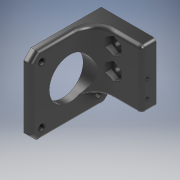
# Autodesk Inventor part: Y-Axis_Motor_Mount_LM3042
Saved by Autodesk Inventor 2020.3 (Build 243373000, 373)
## iProperties
Created: 2020-05-31
Part Number: Y-Axis_Motor_Mount_LM3042
Material: ABS Plastic
Document SubType Name: Modeling
Designer: rah75
Density: 1.06 g/cm^3
Appearance: Satin - Black
Author: rah75
Autodesk Inventor part; units mm, degrees
ref_plane "YZ Plane" through (0, 0, 0) normal (1, 0, 0) x (0, 1, 0)
ref_plane "XZ Plane" through (0, 0, 0) normal (0, 1, 0) x (-1, 0, 0)
ref_plane "XY Plane" through (0, 0, 0) normal (0, 0, 1) x (1, 0, 0)
sketch "Sketch1" plane through (0, 0, 0) normal (0, 0, 1) x (1, 0, 0)
  line L0 (-15, -21.15) -> (15, -21.15)
  line L1 (15, -21.15) -> (15, 21.15)
  line L2 (15, 21.15) -> (-15, 21.15)
  line L3 (-15, 21.15) -> (-15, -21.15)
  line L4 (-15, -21.15) -> (15, 21.15) construction
  line L5 (15, -21.15) -> (-15, 21.15) construction
  point P0 (0, 0)
  dimension "d0" = 30
  dimension "d1" = 42.3
  constraints: 12 end point, 2 midpoint, 2 parallel, 1 horizontal, 1 perpendicular
  measures "d0" distance of L2.end L1.end
  measures "d1" distance of L1.end L0.end
extrude "Extrusion1" add sketch "Sketch1" along normal blind 42.3
sketch "Sketch2" plane through (-15, 21.15, 0) normal (0, 1, 0) x (1, 0, 0)
  line L0 (30, 0) -> (0, 0) projected
  line L1 (0, 0) -> (0, -42.3) projected
  line L2 (30, -42.3) -> (0, -42.3) projected
  line L3 (30, 0) -> (30, -42.3) projected
  line L4 (4, -8) -> (30, -8)
  line L5 (30, -8) -> (30, -42.3)
  line L6 (30, -42.3) -> (4, -42.3)
  line L7 (4, -42.3) -> (4, -8)
  line L8 (4, -8) -> (30, -42.3) construction
  line L9 (30, -8) -> (4, -42.3) construction
  line L10 (30, 0) -> (30, -42.3) projected
  line L11 (30, -42.3) -> (0, -42.3) projected
  point P0 (15, 0)
  point P1 (17, -25.15)
  point P2 (4, -42.3)
  dimension "d4" = 8
  dimension "d5" = 4
  constraints: 12 end point, 2 collinear, 2 midpoint, 2 parallel, 1 horizontal, 1 perpendicular
  measures "d4" distance between parallel lines of L4 L0
  measures "d5" distance between parallel lines of L1 L7
extrude "Extrusion2" cut sketch "Sketch2" against normal through all contours L3 L2 L7 L4
sketch "Sketch3" plane through (-15, -21.15, 0) normal (-1, 0, 0) x (0, 0, 1)
  circle A0 centre (21.15, 21.15) radius 11.25
  line L0 (0, 42.3) -> (0, 0) projected
  line L1 (0, 42.3) -> (42.3, 42.3) projected
  point P0 (0, 21.15)
  point P1 (0, 21.15)
  point P2 (21.15, 42.3)
  dimension "d8" = 22.5
  constraints: 2 midpoint, 1 centre point, 1 horizontal alignment, 1 vertical alignment
  measures "d8" diameter of A0
extrude "Extrusion3" cut sketch "Sketch3" against normal blind 10
sketch "Sketch4" plane through (-11, 21.15, 42.3) normal (1, 0, 0) x (0, 0, -1)
  line L0 (5.65, -36.65) -> (36.65, -36.65) construction
  line L1 (36.65, -36.65) -> (36.65, -5.65) construction
  line L2 (36.65, -5.65) -> (5.65, -5.65) construction
  line L3 (5.65, -5.65) -> (5.65, -36.65) construction
  circle A0 centre (21.15, -21.15) radius 11.25 construction
  line L4 (5.65, -36.65) -> (36.65, -5.65) construction
  line L5 (36.65, -36.65) -> (5.65, -5.65) construction
  point P0 (42.3, -21.15)
  dimension "d11" = 31
  dimension "d12" = 31
  constraints: 12 end point, 4 coincident, 2 midpoint, 2 parallel, 1 horizontal, 1 perpendicular
  measures "d11" distance of L2.end L1.end
  measures "d12" distance of L1.end L0.end
hole "Hole1" at (-11, 15.5, 36.65) at (-11, -15.5, 36.65) at (-11, -15.5, 5.65) direction (-1, 0, 0) diameter 3.4 end through all start extended yes clearance for "Socket Head Cap Screw" size "M3" standard "Ansi Metric M Profile"
sketch "Sketch5" plane through (-11, 21.15, 8) normal (0, 0, 1) x (1, 0, 0)
  line L0 (0, 0) -> (0, -42.3) projected
  line L1 (26, -42.3) -> (0, -42.3) projected
  line L2 (26, 0) -> (26, -42.3) projected
  line L3 (0, -32.3) -> (26, -32.3)
  line L4 (26, -32.3) -> (26, -42.3)
  line L5 (26, -42.3) -> (0, -42.3)
  line L6 (0, -42.3) -> (0, -32.3)
  line L7 (0, -32.3) -> (26, -42.3) construction
  line L8 (26, -32.3) -> (0, -42.3) construction
  line L9 (0, 0) -> (26, 0) projected
  point P0 (11, -21.15)
  point P1 (13, -37.3)
  point P2 (0, -32.3)
  dimension "d21" = 10
  constraints: 12 end point, 2 midpoint, 2 parallel, 1 horizontal, 1 perpendicular
  measures "d21" distance between parallel lines of L3 L1
extrude "Extrusion4" cut sketch "Sketch5" against normal blind 10 contours L3 L2 L1 L0
fillet "Fillet2" radius 10 1 edges at (-11, 5, 8)
chamfer "Chamfer1" distance 4 angle 45 3 edges at (-13, 21.15, 42.3) (-13, -21.15, 42.3) (-13, -21.15, 0)
sketch "Sketch6" plane through (15, -11.15, 8) normal (0, 0, 1) x (1, 0, 0)
  line L0 (4.601, 32.6196) -> (1.0678, 32.6196)
  line L1 (1.0678, 32.6196) -> (1.0678, 6.6196)
  line L2 (1.0678, 6.6196) -> (4.601, 6.6196)
  line L3 (4.601, 6.6196) -> (4.601, 32.6196)
  line L4 (-16, 32.3) -> (0, 32.3) projected
  line L5 (-26, -6) -> (-26, 28.3) projected
  line L6 (-26, -10) -> (-26, -6) projected
  line L7 (0, 32.3) -> (0, 0) projected
  line L8 (-11.125, 22.9184) -> (-15.25, 20.5369)
  line L9 (-15.25, 20.5369) -> (-19.375, 22.9184)
  line L10 (-19.375, 22.9184) -> (-19.375, 27.6816)
  line L11 (-19.375, 27.6816) -> (-15.25, 30.0631)
  line L12 (-15.25, 30.0631) -> (-11.125, 27.6816)
  line L13 (-11.125, 27.6816) -> (-11.125, 22.9184)
  line L14 (-11.125, 10.9184) -> (-15.25, 8.5369)
  line L15 (-15.25, 8.5369) -> (-19.375, 10.9184)
  line L16 (-19.375, 10.9184) -> (-19.375, 15.6816)
  line L17 (-19.375, 15.6816) -> (-15.25, 18.0631)
  line L18 (-15.25, 18.0631) -> (-11.125, 15.6816)
  line L19 (-11.125, 15.6816) -> (-11.125, 10.9184)
  line L20 (-30, 28.3) -> (-30, -6) projected
  point P0 (-15, 11.15)
  point P1 (-15.25, 25.3)
  point P2 (-15.25, 13.3)
  point P3 (-15.25, 25.3)
  point P4 (-15.25, 13.3)
  dimension "d29" = 26
  dimension "d30" = 7
  dimension "d31" = 19
  dimension "d33" = 8.25
  dimension "d45" = 14.75
  constraints: 32 end point, 2 coincident, 2 parallel, 1 collinear, 1 horizontal, 1 perpendicular, 1 point on line, 1 vertical, 1 vertical alignment, 26 other
  measures "d29" distance of L1.end L0.end
  measures "d30" distance from line of L4 point (-15.25, 25.3)
  measures "d31" distance from line of L4 point (-15.25, 13.3)
  measures "d33" distance between parallel lines of L16 L19
  measures "d45" distance from line of L20 point (-15.25, 25.3)
extrude "Extrusion5" cut sketch "Sketch6" along normal blind 10 and the other way blind 3 contours L8 L9 L10 L11 L12 L13 | L14 L15 L16 L17 L18 L19
hole "Hole2" at (-0.25, 14.15, 8) at (-0.25, 2.15, 8) direction (0, 0, -1) diameter 5.5 end through all start extended yes clearance for "Socket Head Cap Screw" size "M5" standard "Ansi Metric M Profile"
fillet "Fillet3" radius 2 12 edges at (-11, 21.15, 28.15) (7, 21.15, 8) (-8.0711, 21.15, 10.9289) (15, 21.15, 4) (15, 5, 8) (15, -11.15, 4) (-8.0711, -11.15, 10.9289) (7, -11.15, 8) (-11, 19.15, 40.3) (-11, 0, 42.3) (-11, -19.15, 40.3) (-11, -21.15, 21.15)
sketch "Sketch7" plane through (15, -17.15, 0) normal (1, 0, 0) x (0, 0, -1)
  line L0 (-5, 21.9) -> (-5, 12.4) construction
  line L1 (-42.3, 34.3) -> (-42.3, 0) projected
  line L2 (0, 8) -> (0, 36.3) projected
  point P0 (0, 17.15)
  point P1 (-5, 17.15)
  dimension "d46" = 9.5
  dimension "d55" = 5
  constraints: 2 coincident, 2 end point, 1 horizontal alignment, 1 midpoint, 1 vertical
  measures "d46" distance of L0.start L0.end
  measures "d55" distance between parallel lines of L2 L0
hole "Hole3" at (15, 4.75, 5) at (15, -4.75, 5) direction (-1, 0, 0) diameter 1.75 depth 9.5 tip angle 118
body "Solid1"
